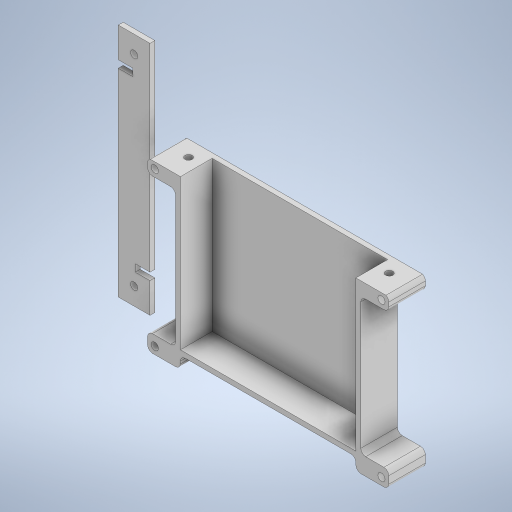
# Autodesk Inventor part: Caixa_baterias_em_baixo
Saved by Autodesk Inventor 2024 (Build 280153000, 153)
## iProperties
Created: 2023-05-26
Part Number: Caixa_baterias_em_baixo
Material: Generic
Document SubType Name: Modeling
Designer: guilh
Density: 1 g/cm^3
Appearance: Default
Author: guilh
Autodesk Inventor part; units mm, degrees
ref_plane "YZ Plane" through (0, 0, 0) normal (1, 0, 0) x (0, 1, 0)
ref_plane "XZ Plane" through (0, 0, 0) normal (0, 1, 0) x (-1, 0, 0)
ref_plane "XY Plane" through (0, 0, 0) normal (0, 0, 1) x (1, 0, 0)
sketch "Sketch1" plane through (0, 0, 0) normal (0, 0, 1) x (1, 0, 0)
  arc A0 (-97.827, 68.5405) -> (-99, 66.7195) centre (-97, 66.7195) ccw
  arc A1 (0, 66.7195) -> (-1.173, 68.5405) centre (-2, 66.7195) ccw
  arc A2 (-99, 2) -> (-97, 0) centre (-97, 2) ccw
  arc A3 (-2, 0) -> (0, 2) centre (-2, 2) ccw
  circle A4 centre (-3, 3) radius 1.5
  circle A5 centre (-96, 3) radius 1.5
  circle A6 centre (-3, 66) radius 1.5
  circle A7 centre (-96, 66) radius 1.5
  line L0 (-97.827, 68.5405) -> (-1.173, 68.5405)
  line L1 (-64.75, 66) -> (-34.25, 66)
  line L2 (-64.75, 66) -> (-64.75, 42.5)
  line L3 (-64.75, 42.5) -> (-34.25, 42.5)
  line L4 (-34.25, 42.5) -> (-34.25, 66)
  line L5 (-83.5, 5) -> (-15.5, 5)
  line L6 (-11.5, 9) -> (-11.5, 61)
  line L7 (-87.5, 9) -> (-87.5, 61)
  line L8 (-89.5, 63) -> (-97, 63)
  line L9 (-89.5, 7) -> (-97, 7)
  line L10 (-85.5, 3) -> (-85.5, 2)
  line L11 (-11.5, 9) -> (-11.5, 61)
  line L12 (-9.5, 63) -> (-2, 63)
  line L13 (-9.5, 7) -> (-2, 7)
  line L14 (-13.5, 3) -> (-13.5, 2)
  line L15 (-99, 2) -> (-99, 5)
  line L16 (-99, 65) -> (-99, 66.7195)
  line L17 (0, 2) -> (0, 5)
  line L18 (0, 65) -> (0, 66.7195)
  line L19 (-2, 0) -> (-11.5, 0)
  line L20 (-87.5, 0) -> (-97, 0)
  arc A8 (-87.5, 61) -> (-89.5, 63) centre (-89.5, 61) ccw
  arc A9 (-9.5, 63) -> (-11.5, 61) centre (-9.5, 61) ccw
  arc A10 (-11.5, 9) -> (-9.5, 7) centre (-9.5, 9) ccw
  arc A11 (-13.5, 3) -> (-15.5, 5) centre (-15.5, 3) ccw
  arc A12 (-83.5, 5) -> (-85.5, 3) centre (-83.5, 3) ccw
  arc A13 (-89.5, 7) -> (-87.5, 9) centre (-89.5, 9) ccw
  arc A14 (-2, 63) -> (0, 65) centre (-2, 65) ccw
  arc A15 (-99, 65) -> (-97, 63) centre (-97, 65) ccw
  arc A16 (-97, 7) -> (-99, 5) centre (-97, 5) ccw
  arc A17 (-87.5, 0) -> (-85.5, 2) centre (-87.5, 2) ccw
  arc A18 (-13.5, 2) -> (-11.5, 0) centre (-11.5, 2) ccw
  arc A19 (0, 5) -> (-2, 7) centre (-2, 5) ccw
  point P0 (0, 0)
  point P1 (-99, 68)
  point P2 (-97, 2)
  point P3 (-85.5, 5)
  point P4 (-87.5, 63)
  point P5 (-99, 63)
  point P6 (-99, 7)
  point P7 (-85.5, 0)
  point P8 (-87.5, 7)
  point P9 (0, 63)
  point P10 (0, 7)
  point P11 (-13.5, 0)
  point P12 (-13.5, 5)
  dimension "d5" = 2
  dimension "d6" = 2
  dimension "d7" = 2
  dimension "d8" = 2
  dimension "d14" = 3
  dimension "d16" = 3
  dimension "d94" = 3
  dimension "d95" = 3
  dimension "d97" = 99
  dimension "d98" = 30.5
  dimension "d99" = 23.5
  dimension "d190" = 96.654
  dimension "d200" = 10.327
  dimension "d228" = 2
  dimension "d229" = 2
  dimension "d230" = 2
  constraints: 42 end point, 36 tangent, 32 point on circle, 20 centre point, 20 point on line, 13 perpendicular, 9 equal radius, 4 horizontal, 4 vertical, 1 coincident
  measures "d5" radius of A0
  measures "d6" radius of A1
  measures "d7" radius of A2
  measures "d8" radius of A3
  measures "d14" diameter of A4
  measures "d16" diameter of A6
  measures "d94" diameter of A7
  measures "d95" diameter of A5
  measures "d97" distance of L18.end L16.end
  measures "d98" distance of L1.start L1.end
  measures "d99" distance of L1.start L2.end
  measures "d190" distance of L0.end L0.start
  measures "d200" horizontal distance of L0.end L6.end
  measures "d228" radius of A8
  measures "d229" radius of A9
  measures "d230" radius of A16
extrude "Extrusion1" add sketch "Sketch1" against normal blind 2 contours L0 A1 L18 A14 L12 A9 L6 A10 L13 A19 L17 A3 L19 A18 L14 A11 L5 A12 L10 A17 L20 A2 L15 A16 L9 A13 L7 A8 L8 A15 L16 A0 | L1 L4 L3 L2
sketch "Sketch2" plane through (0, 0, 0) normal (0, 0, 1) x (1, 0, 0)
  arc A0 (-97.827, 68.5405) -> (-99, 66.7195) centre (-97, 66.7195) ccw
  arc A1 (0, 66.7195) -> (-1.173, 68.5405) centre (-2, 66.7195) ccw
  arc A2 (-99, 2) -> (-97, 0) centre (-97, 2) ccw
  arc A3 (-2, 0) -> (0, 2) centre (-2, 2) ccw
  circle A4 centre (-3, 3) radius 1.5
  circle A5 centre (-96, 3) radius 1.5
  circle A6 centre (-3, 66) radius 1.5
  circle A7 centre (-96, 66) radius 1.5
  line L0 (-97.827, 68.5405) -> (-1.173, 68.5405)
  line L1 (-64.75, 66) -> (-34.25, 66)
  line L2 (-64.75, 66) -> (-64.75, 42.5)
  line L3 (-64.75, 42.5) -> (-34.25, 42.5)
  line L4 (-34.25, 42.5) -> (-34.25, 66)
  line L5 (-83.5, 5) -> (-15.5, 5)
  line L6 (-11.5, 9) -> (-11.5, 61)
  line L7 (-87.5, 9) -> (-87.5, 61)
  line L8 (-89.5, 63) -> (-97, 63)
  line L9 (-89.5, 7) -> (-97, 7)
  line L10 (-85.5, 3) -> (-85.5, 2)
  line L11 (-13.5, 3) -> (-13.5, 2)
  line L12 (-11.5, 9) -> (-11.5, 61)
  line L13 (-9.5, 7) -> (-2, 7)
  line L14 (-9.5, 63) -> (-2, 63)
  line L15 (-99, 2) -> (-99, 5)
  line L16 (-99, 65) -> (-99, 66.7195)
  line L17 (0, 2) -> (0, 5)
  line L18 (0, 65) -> (0, 66.7195)
  line L19 (-2, 0) -> (-11.5, 0)
  line L20 (-87.5, 0) -> (-97, 0)
  arc A8 (-87.5, 61) -> (-89.5, 63) centre (-89.5, 61) ccw
  arc A9 (-9.5, 63) -> (-11.5, 61) centre (-9.5, 61) ccw
  arc A10 (-11.5, 9) -> (-9.5, 7) centre (-9.5, 9) ccw
  arc A11 (-13.5, 3) -> (-15.5, 5) centre (-15.5, 3) ccw
  arc A12 (-83.5, 5) -> (-85.5, 3) centre (-83.5, 3) ccw
  arc A13 (-89.5, 7) -> (-87.5, 9) centre (-89.5, 9) ccw
  arc A14 (-2, 63) -> (0, 65) centre (-2, 65) ccw
  arc A15 (-99, 65) -> (-97, 63) centre (-97, 65) ccw
  arc A16 (-97, 7) -> (-99, 5) centre (-97, 5) ccw
  arc A17 (-87.5, 0) -> (-85.5, 2) centre (-87.5, 2) ccw
  arc A18 (-13.5, 2) -> (-11.5, 0) centre (-11.5, 2) ccw
  arc A19 (0, 5) -> (-2, 7) centre (-2, 5) ccw
  line L21 (-85.5, 68.5405) -> (-85.5, 7)
  line L22 (-85.5, 7) -> (-13.5, 7)
  line L23 (-13.5, 7) -> (-13.5, 68.5405)
  point P0 (0, 0)
  point P1 (-99, 68)
  point P2 (-97, 2)
  point P3 (-85.5, 5)
  point P4 (-87.5, 63)
  point P5 (-99, 63)
  point P6 (-99, 7)
  point P7 (-85.5, 0)
  point P8 (-87.5, 7)
  point P9 (-13.5, 0)
  point P10 (0, 7)
  point P11 (0, 63)
  point P12 (-13.5, 5)
  point P13 (-89.5, 7)
  dimension "d231" = 2
  dimension "d232" = 2
  dimension "d233" = 2
  dimension "d234" = 2
  dimension "d235" = 3
  dimension "d236" = 3
  dimension "d237" = 3
  dimension "d238" = 3
  dimension "d239" = 99
  dimension "d240" = 30.5
  dimension "d241" = 23.5
  dimension "d242" = 96.654
  dimension "d243" = 10.327
  dimension "d244" = 2
  dimension "d245" = 2
  dimension "d246" = 2
  constraints: 48 end point, 36 tangent, 32 point on circle, 22 point on line, 20 centre point, 14 perpendicular, 9 equal radius, 5 vertical, 4 horizontal, 1 coincident
  measures "d231" radius of A0
  measures "d232" radius of A1
  measures "d233" radius of A2
  measures "d234" radius of A3
  measures "d235" diameter of A4
  measures "d236" diameter of A6
  measures "d237" diameter of A7
  measures "d238" diameter of A5
  measures "d239" distance of L18.end L16.end
  measures "d240" distance of L1.start L1.end
  measures "d241" distance of L1.start L3.start
  measures "d242" distance of L0.end L0.start
  measures "d243" horizontal distance of L0.end L6.end
  measures "d244" radius of A8
  measures "d245" radius of A9
  measures "d246" radius of A16
extrude "Extrusion2" add sketch "Sketch2" along normal blind 13 contours L0 L21 L22 L23 A1 L18 A14 L14 A9 L6 A10 L13 A19 L17 A3 L19 A18 L11 A11 L5 A12 L10 A17 L20 A2 L15 A16 L9 A13 L7 A8 L8 A15 L16 A0
sketch "Sketch3" plane through (0, 0, 0) normal (0, 0, 1) x (1, 0, 0)
  line L0 (-117, 15.327) -> (-111, 15.327)
  line L1 (-117, 12.327) -> (-117, 15.327)
  line L2 (-111, 12.327) -> (-117, 12.327)
  line L3 (-118, 81.327) -> (-124, 81.327)
  line L4 (-124, 84.327) -> (-118, 84.327)
  line L5 (-118, 84.327) -> (-118, 81.327)
  line L6 (-118, 81.327) -> (-124, 81.327)
  line L7 (-111, 0) -> (-111, 12.327)
  line L8 (-111, 15.327) -> (-111, 96.654)
  line L9 (-124, 84.327) -> (-124, 96.654)
  line L10 (-124, 81.327) -> (-124, 0)
  line L11 (-111, 96.654) -> (-124, 96.654)
  line L12 (-124, 0) -> (-111, 0)
  point P0 (0, 0)
  point P1 (-111, 0)
  dimension "d194" = 6
  dimension "d195" = 3
  dimension "d201" = 12.327
  dimension "d227" = 13
  constraints: 26 end point, 3 perpendicular, 2 vertical, 1 horizontal, 1 parallel
  measures "d194" distance of L2.start L1.start
  measures "d195" distance of L1.start L0.start
  measures "d201" distance of L7.start L7.end
  measures "d227" distance of L8.end L11.end
sketch "Sketch4" plane through (0, 0, -2) normal (0, 0, -1) x (-1, 0, 0)
  arc A0 (1.173, 68.5405) -> (0, 66.7195) centre (2, 66.7195) ccw
  arc A1 (99, 66.7195) -> (97.827, 68.5405) centre (97, 66.7195) ccw
  arc A2 (0, 2) -> (2, 0) centre (2, 2) ccw
  arc A3 (97, 0) -> (99, 2) centre (97, 2) ccw
  circle A4 centre (96, 3) radius 1.5
  circle A5 centre (3, 3) radius 1.5
  circle A6 centre (96, 66) radius 1.5
  circle A7 centre (3, 66) radius 1.5
  line L0 (1.173, 68.5405) -> (97.827, 68.5405)
  line L1 (34.25, 66) -> (64.75, 66)
  line L2 (34.25, 66) -> (34.25, 42.5)
  line L3 (34.25, 42.5) -> (64.75, 42.5)
  line L4 (64.75, 42.5) -> (64.75, 66)
  line L5 (13.5, 5) -> (85.5, 5)
  line L6 (87.5, 7) -> (87.5, 63)
  line L7 (11.5, 7) -> (11.5, 63)
  line L8 (11.5, 63) -> (0, 63)
  line L9 (11.5, 7) -> (0, 7)
  line L10 (13.5, 5) -> (13.5, 0)
  line L11 (85.5, 5) -> (85.5, 0)
  line L12 (87.5, 7) -> (87.5, 63)
  line L13 (87.5, 7) -> (99, 7)
  line L14 (87.5, 63) -> (99, 63)
  line L15 (0, 2) -> (0, 7)
  line L16 (0, 63) -> (0, 66.7195)
  line L17 (99, 2) -> (99, 7)
  line L18 (99, 63) -> (99, 66.7195)
  line L19 (97, 0) -> (85.5, 0)
  line L20 (13.5, 0) -> (2, 0)
  line L21 (65.25, 42) -> (33.75, 42)
  line L22 (33.75, 42) -> (33.75, 66.5)
  line L23 (33.75, 66.5) -> (65.25, 66.5)
  line L24 (65.25, 42) -> (65.25, 66.5)
  point P0 (0, 0)
  point P1 (99, 0)
  point P2 (0, 68)
  point P3 (2, 2)
  dimension "d140" = 2
  dimension "d141" = 2
  dimension "d143" = 2
  dimension "d144" = 3
  dimension "d145" = 3
  dimension "d146" = 3
  dimension "d147" = 3
  dimension "d148" = 99
  dimension "d149" = 30.5
  dimension "d150" = 23.5
  dimension "d151" = 0.5
  constraints: 50 end point, 14 perpendicular, 12 tangent, 8 centre point, 8 point on circle, 5 horizontal, 4 vertical, 1 coincident, 1 parallel, 1 other
  measures "d140" radius of A0
  measures "d141" radius of A1
  measures "d143" radius of A3
  measures "d144" diameter of A4
  measures "d145" diameter of A6
  measures "d146" diameter of A7
  measures "d147" diameter of A5
  measures "d148" distance of L18.end L16.end
  measures "d149" distance of L2.start L1.end
  measures "d150" distance of L2.start L2.end
  measures "d151" distance between parallel lines of L2 L22
extrude "Extrusion4" cut sketch "Sketch4" against normal blind 0.5 contours L21 L22 L23 L24
extrude "Extrusion3" add sketch "Sketch3" against normal blind 2
sketch "Sketch5" plane through (-97.827, 68.5405, -2) normal (0, 1, 0) x (1, 0, 0)
  circle A0 centre (89.4905, -6.5) radius 1.5
  circle A1 centre (7.1635, -6.5) radius 1.5
  point P0 (97.827, -2)
  constraints: 2 centre point
extrude "Extrusion5" cut sketch "Sketch5" against normal blind 6
sketch "Sketch6" plane through (0, 0, 0) normal (0, 0, 1) x (1, 0, 0)
  line L0 (-117.5, 87.327) -> (-117.5, 87.327)
  circle A0 centre (-117.5, 89.4905) radius 1.5
  circle A1 centre (-117.5, 7.1635) radius 1.5
  point P0 (0, 0)
  point P1 (-116.5, 87.327)
  point P2 (-118.5, 87.327)
  dimension "d222" = 2
  constraints: 2 centre point, 2 end point, 2 point on line
  measures "d222" distance of point (-116.5, 87.327) point (-118.5, 87.327)
extrude "Extrusion6" cut sketch "Sketch6" against normal blind 2
body "Solid1"
